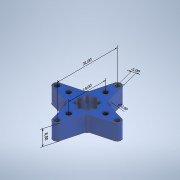
# Autodesk Inventor part: servo horn
Saved by Autodesk Inventor 2022 (Build 260153000, 153)
## iProperties
Created: 2021-02-24
Part Number: servo horn
Material: Titanium
Document SubType Name: Modeling
Designer: WASHINGTON
Density: 4.51 g/cm^3
Appearance: Titanium
Author: WASHINGTON
Autodesk Inventor part; units mm, degrees
ref_plane "YZ Plane" through (0, 0, 0) normal (1, 0, 0) x (0, 1, 0)
ref_plane "XZ Plane" through (0, 0, 0) normal (0, 1, 0) x (-1, 0, 0)
ref_plane "XY Plane" through (0, 0, 0) normal (0, 0, 1) x (1, 0, 0)
sketch "Sketch1" plane through (0, 0, 0) normal (0, 1, 0) x (-1, 0, 0)
  circle A0 centre (0, 0) radius 4
  line L0 (4, 0) -> (5, 0) construction
  line L1 (5, 0) -> (5, -0.5)
  line L2 (5, -0.5) -> (3.8219, -1.1802)
  line L3 (5, 0) -> (5, 0.5)
  line L4 (5, 0.5) -> (3.8219, 1.1802)
  line L5 (3.8891, 3.182) -> (3.537, 1.868)
  line L6 (3.5355, 3.5355) -> (3.8891, 3.182)
  line L7 (3.5355, 3.5355) -> (3.182, 3.8891)
  line L8 (3.182, 3.8891) -> (1.868, 3.537)
  line L9 (0.5, 5) -> (1.1802, 3.8219)
  line L10 (0, 5) -> (0.5, 5)
  line L11 (0, 5) -> (-0.5, 5)
  line L12 (-0.5, 5) -> (-1.1802, 3.8219)
  line L13 (-3.182, 3.8891) -> (-1.868, 3.537)
  line L14 (-3.5355, 3.5355) -> (-3.182, 3.8891)
  line L15 (-3.5355, 3.5355) -> (-3.8891, 3.182)
  line L16 (-3.8891, 3.182) -> (-3.537, 1.868)
  line L17 (-5, 0.5) -> (-3.8219, 1.1802)
  line L18 (-5, 0) -> (-5, 0.5)
  line L19 (-5, 0) -> (-5, -0.5)
  line L20 (-5, -0.5) -> (-3.8219, -1.1802)
  line L21 (-3.8891, -3.182) -> (-3.537, -1.868)
  line L22 (-3.5355, -3.5355) -> (-3.8891, -3.182)
  line L23 (-3.5355, -3.5355) -> (-3.182, -3.8891)
  line L24 (-3.182, -3.8891) -> (-1.868, -3.537)
  line L25 (-0.5, -5) -> (-1.1802, -3.8219)
  line L26 (0, -5) -> (-0.5, -5)
  line L27 (0, -5) -> (0.5, -5)
  line L28 (0.5, -5) -> (1.1802, -3.8219)
  line L29 (3.182, -3.8891) -> (1.868, -3.537)
  line L30 (3.5355, -3.5355) -> (3.182, -3.8891)
  line L31 (3.5355, -3.5355) -> (3.8891, -3.182)
  line L32 (3.8891, -3.182) -> (3.537, -1.868)
  circle A1 centre (0, 0) radius 17.5 construction
  arc A2 (15.5, -2) -> (15.5, 2) centre (15.5, 0) ccw
  line L33 (15.5, 2) -> (0, 2) construction
  line L34 (15.5, -2) -> (0, -2) construction
  line L35 (16.0176, 1.9319) -> (5.8875, 4.6462)
  line L36 (20.0758, 0) -> (0, 0) construction
  line L37 (16.0176, -1.9319) -> (5.8875, -4.6462)
  line L38 (-1.9319, 16.0176) -> (-4.6462, 5.8875)
  line L39 (1.9319, 16.0176) -> (4.6462, 5.8875)
  arc A3 (2, 15.5) -> (-2, 15.5) centre (0, 15.5) ccw
  line L40 (-16.0176, -1.9319) -> (-5.8875, -4.6462)
  line L41 (-16.0176, 1.9319) -> (-5.8875, 4.6462)
  arc A4 (-15.5, 2) -> (-15.5, -2) centre (-15.5, 0) ccw
  line L42 (1.9319, -16.0176) -> (4.6462, -5.8875)
  line L43 (-1.9319, -16.0176) -> (-4.6462, -5.8875)
  arc A5 (-2, -15.5) -> (2, -15.5) centre (0, -15.5) ccw
  arc A6 (5.8875, 4.6462) -> (4.6462, 5.8875) centre (0, 0) ccw
  arc A7 (-4.6462, 5.8875) -> (-5.8875, 4.6462) centre (0, 0) ccw
  arc A8 (-5.8875, -4.6462) -> (-4.6462, -5.8875) centre (0, 0) ccw
  arc A9 (4.6462, -5.8875) -> (5.8875, -4.6462) centre (0, 0) ccw
  circle A10 centre (0, 15.5) radius 1.25
  circle A11 centre (0, 9.5) radius 1.25
  circle A12 centre (-9.5, 0) radius 1.25
  circle A13 centre (-15.5, 0) radius 1.25
  circle A14 centre (0, -9.5) radius 1.25
  circle A15 centre (0, -15.5) radius 1.25
  circle A16 centre (9.5, 0) radius 1.25
  circle A17 centre (15.5, 0) radius 1.25
  point P0 (-3.8219, -1.1802)
  point P1 (-3.8219, 1.1802)
  dimension "d0" = 8
  dimension "d1" = 120
  dimension "d2" = 1
  dimension "d3" = 0.5
  dimension "d4" = 5
  dimension "d7" = 360
  dimension "d9" = 35
  dimension "d11" = 4
  dimension "d14" = 15
  dimension "d15" = 0
  dimension "d18" = 360
  dimension "d20" = 7.5
  dimension "d21" = 0.8157
  dimension "d22" = 4.0798
  dimension "d23" = 7.9436
  dimension "d24" = 2.5
  dimension "d25" = 2.5
  dimension "d26" = 6
  dimension "d27" = 9.5
  dimension "d30" = 360
  constraints: 88 end point, 22 point on circle, 18 centre point, 4 coincident, 4 horizontal, 4 symmetric about line, 4 tangent, 1 perpendicular, 131 other
  measures "d0" diameter of A0
  measures "d1" angle of L2 L1
  measures "d2" distance of L0.start L0.end
  measures "d3" distance of L0.end L1.end
  measures "d4" distance of point (0, 0) L0.end
  measures "d9" diameter of A1
  measures "d11" diameter of A2
  measures "d14" angle of L33 L35
  measures "d15" vertical distance of point (0, 0) A2.centre
  measures "d20" radius of A9
  measures "d21" distance from line of L36.start L35
  measures "d22" distance from line of L33.end L35
  measures "d23" distance from line of L34.end L35
  measures "d24" diameter of A10
  measures "d25" diameter of A11
  measures "d26" distance of A3.centre A11.centre
  measures "d27" distance of point (0, 0) A11.centre
extrude "Extrusion1" add sketch "Sketch1" along normal mid plane 8
thread "Thread1" size "M2.5x0.45" class "6H" standard "ANSI Metric M Profile" full length
thread "Thread2" size "M2.5x0.45" class "6H" standard "ANSI Metric M Profile" full length
thread "Thread3" size "M2.5x0.45" class "6H" standard "ANSI Metric M Profile" full length
thread "Thread4" size "M2.5x0.45" class "6H" standard "ANSI Metric M Profile" full length
thread "Thread5" size "M2.5x0.45" class "6H" standard "ANSI Metric M Profile" full length
thread "Thread6" size "M2.5x0.45" class "6H" standard "ANSI Metric M Profile" full length
thread "Thread7" size "M2.5x0.45" class "6H" standard "ANSI Metric M Profile" full length
thread "Thread8" size "M2.5x0.45" class "6H" standard "ANSI Metric M Profile" full length
thread "Thread9" size "M2.5x0.45" class "6H" standard "ANSI Metric M Profile" full length
body "Solid1"
